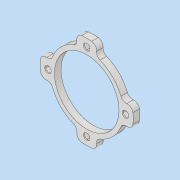
# Autodesk Inventor part: MotorMountNutHolder
Saved by Autodesk Inventor 2017.3 (Build 213256000, 256)
## iProperties
Created: 2018-12-18
Part Number: MotorMountNutHolder
Material: ABS Plastic
Document SubType Name: Modeling
Designer: Derek Wider
Density: 1.06 g/cm^3
Appearance: Smooth - White
Author: Derek Wider
Autodesk Inventor part; units mm, degrees
ref_plane "YZ Plane" through (0, 0, 0) normal (1, 0, 0) x (0, 1, 0)
ref_plane "XZ Plane" through (0, 0, 0) normal (0, 1, 0) x (-1, 0, 0)
ref_plane "XY Plane" through (0, 0, 0) normal (0, 0, 1) x (1, 0, 0)
sketch "Sketch1" plane through (0, 0, 0) normal (0, 0, 1) x (1, 0, 0)
  circle A0 centre (0, 0) radius 18.7325
  circle A1 centre (0, 0) radius 26.9875
  dimension "d0" = 37.465
  dimension "d1" = 53.975
  constraints: 2 centre point, 2 coincident
  measures "d0" diameter of A0
  measures "d1" diameter of A1
extrude "Extrusion1" add sketch "Sketch1" along normal blind 3.81
sketch "Sketch2" plane through (0, 0, 0) normal (0, 0, -1) x (-1, 0, 0)
  line L0 (-1.9431, 19.1389) -> (-3.8861, 22.5044)
  line L1 (-3.8861, 22.5044) -> (-1.9431, 25.8699)
  line L2 (-1.9431, 25.8699) -> (1.9431, 25.8699)
  line L3 (1.9431, 25.8699) -> (3.8861, 22.5044)
  line L4 (3.8861, 22.5044) -> (1.9431, 19.1389)
  line L5 (1.9431, 19.1389) -> (-1.9431, 19.1389)
  point P0 (0, 0)
  point P1 (0, 22.5044)
  dimension "d4" = 22.5044
  dimension "d5" = 6.731
  constraints: 12 end point, 1 horizontal, 1 vertical alignment, 13 other
  measures "d4" distance of point (0, 0) point (0, 22.504)
  measures "d5" distance between parallel lines of L5 L2
extrude "Extrusion2" cut sketch "Sketch2" against normal blind 3.175
sketch "Sketch3" plane through (0, 0, 3.175) normal (0, 0, -1) x (-1, 0, 0)
  line L0 (-1.9431, 19.1389) -> (-3.8861, 22.5044) construction
  line L1 (1.9431, 19.1389) -> (-1.9431, 19.1389) construction
  line L2 (3.8861, 22.5044) -> (1.9431, 19.1389) construction
  line L3 (1.9431, 25.8699) -> (3.8861, 22.5044) construction
  line L4 (-1.9431, 25.8699) -> (1.9431, 25.8699) construction
  line L5 (-3.8861, 22.5044) -> (-1.9431, 25.8699) construction
  circle A0 centre (0, 22.5044) radius 1.905
  point P0 (0, 0)
  dimension "d8" = 3.81
  constraints: 1 centre point, 1 horizontal alignment
  measures "d8" diameter of A0
extrude "Extrusion3" cut sketch "Sketch3" against normal blind 3.175
pattern_circular "Circular Pattern1" count 4 over 360 about axis through (0, 0, 0) along (0, 0, 1) of "Extrusion3", "Extrusion2"
sketch "Sketch4" plane through (0, 0, 0) normal (0, 0, -1) x (-1, 0, 0)
  arc A0 (-5.08, 20.657) -> (-20.657, 5.08) centre (0, 0) ccw
  line L0 (-5.08, 20.657) -> (-6.4448, 26.2067)
  line L1 (-20.657, 5.08) -> (-26.2067, 6.4448)
  arc A1 (-6.4448, 26.2067) -> (-26.2067, 6.4448) centre (0, 0) ccw
  circle A2 centre (0, 0) radius 26.9875 construction
  dimension "d14" = 42.545
  dimension "d15" = 5.08
  dimension "d16" = 5.08
  constraints: 4 end point, 4 point on circle, 2 centre point, 2 coincident, 2 line through centre, 2 other
  measures "d14" diameter of A0
  measures "d15" horizontal distance of point (0, 0) L0.start
  measures "d16" vertical distance of point (0, 0) L1.start
extrude "Extrusion4" cut sketch "Sketch4" against normal through all
fillet "Fillet1" radius 3.175 4 edges at (6.4448, 26.2067, 1.905) (5.08, 20.657, 1.905) (20.657, 5.08, 1.905) (26.2067, 6.4448, 1.905)
pattern_circular "Circular Pattern2" count 4 over 360 about axis through (0, 0, 0) along (0, 0, 1) of "Extrusion4", "Fillet1"
body "Solid1"
